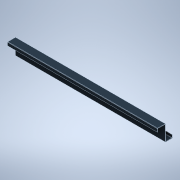
# Autodesk Inventor part: PerfilZ
Saved by Autodesk Inventor 2021 (Build 250183000, 183)
## iProperties
Created: 2021-06-04
Part Number: PerfilZ
Material: Generic
Document SubType Name: Modeling
Designer: Nelson
Density: 1 g/cm^3
Appearance: Default(5)
Author: Nelson
Autodesk Inventor part; units mm, degrees
ref_plane "YZ Plane" through (0, 0, 0) normal (1, 0, 0) x (0, 1, 0)
ref_plane "XZ Plane" through (0, 0, 0) normal (0, 1, 0) x (-1, 0, 0)
ref_plane "XY Plane" through (0, 0, 0) normal (0, 0, 1) x (1, 0, 0)
sketch "Sketch1" plane through (0, 0, 0) normal (1, 0, 0) x (0, 1, 0)
  line L0 (2, 0) -> (102, 0)
  line L1 (0, -2) -> (0, -46)
  line L2 (104, 2) -> (104, 48)
  line L3 (2, -48) -> (20, -48)
  line L4 (102, 50) -> (84, 50)
  line L5 (84, 52.5) -> (104.5, 52.5)
  line L6 (106.5, 50.5) -> (106.5, -0.5)
  line L7 (104.5, -2.5) -> (4.5, -2.5)
  line L8 (2.5, -4.5) -> (2.5, -43.5)
  line L9 (4.5, -45.5) -> (20, -45.5)
  line L10 (84, 52.5) -> (84, 50)
  line L11 (20, -45.5) -> (20, -48)
  arc A0 (104, 48) -> (102, 50) centre (102, 48) ccw
  arc A1 (106.5, 50.5) -> (104.5, 52.5) centre (104.5, 50.5) ccw
  arc A2 (102, 0) -> (104, 2) centre (102, 2) ccw
  arc A3 (104.5, -2.5) -> (106.5, -0.5) centre (104.5, -0.5) ccw
  arc A4 (2, 0) -> (0, -2) centre (2, -2) ccw
  arc A5 (4.5, -2.5) -> (2.5, -4.5) centre (4.5, -4.5) ccw
  arc A6 (2.5, -43.5) -> (4.5, -45.5) centre (4.5, -43.5) ccw
  arc A7 (0, -46) -> (2, -48) centre (2, -46) ccw
  point P0 (0, 0)
  point P1 (104, 0)
  point P2 (0, -48)
  point P3 (104, 50)
  point P4 (106.5, 52.5)
  point P5 (106.5, -2.5)
  point P6 (2.5, -2.5)
  point P7 (2.5, -45.5)
  dimension "d0" = 104
  dimension "d1" = 48
  dimension "d2" = 50
  dimension "d3" = 20
  dimension "d4" = 20
  dimension "d5" = 2.5
  dimension "d8" = 2
  constraints: 24 end point, 16 point on circle, 16 point on line, 16 tangent, 8 centre point, 7 equal radius, 4 vertical, 3 horizontal, 4 other
  measures "d0" distance of point (0, 0) point (104, 0)
  measures "d1" distance of point (0, 0) point (0, -48)
  measures "d2" distance of point (104, 0) point (104, 50)
  measures "d3" distance of point (0, -48) L3.end
  measures "d4" distance of point (104, 50) L4.end
  measures "d5" distance between parallel lines of L4 L5
  measures "d8" radius of A0
extrude "Extrusion1" add sketch "Sketch1" against normal blind 1000
body "Solid1"
